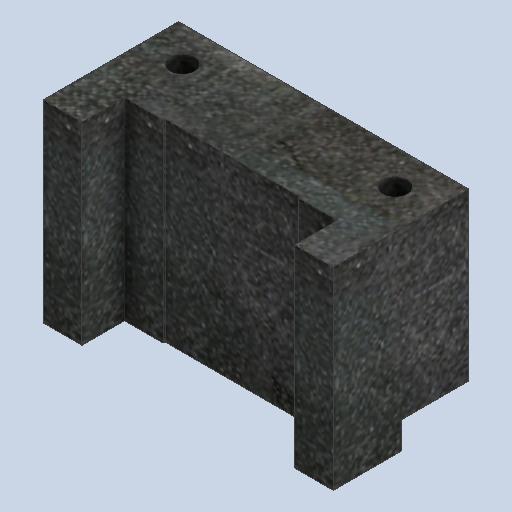
# Autodesk Inventor part: Lose backe
Saved by Autodesk Inventor 2023.2 (Build 272271000, 271)
## iProperties
Created: 2023-02-07
Part Number: Lose backe
Material: Steel
Document SubType Name: Modeling
Designer: Ayush
Density: 7.85 g/cm^3
Appearance: Plate
Author: Ayush
Autodesk Inventor part; units mm, degrees
ref_plane "YZ Plane" through (0, 0, 0) normal (1, 0, 0) x (0, 1, 0)
ref_plane "XZ Plane" through (0, 0, 0) normal (0, 1, 0) x (-1, 0, 0)
ref_plane "XY Plane" through (0, 0, 0) normal (0, 0, 1) x (1, 0, 0)
sketch "Sketch1" plane through (0, 0, 0) normal (0, 1, 0) x (-1, 0, 0)
  line L0 (-37.5, -17.5) -> (37.5, -17.5)
  line L1 (37.5, -17.5) -> (37.5, 17.5)
  line L2 (-37.5, 17.5) -> (-37.5, -17.5)
  line L3 (-37.5, -17.5) -> (37.5, 17.5) construction
  line L4 (37.5, -17.5) -> (-37.5, 17.5) construction
  line L5 (37.5, 17.5) -> (27.5, 17.5)
  line L6 (27.5, 17.5) -> (27.5, 6.5)
  line L7 (27.5, 6.5) -> (17.5, 6.5)
  line L8 (17.5, 6.5) -> (17.5, 6.0228)
  line L9 (17.5, 6.0228) -> (-17.5, 6.0228)
  line L10 (-17.5, 6.0228) -> (-17.5, 6.5)
  line L11 (-17.5, 6.5) -> (-27.5, 6.5)
  line L12 (-27.5, 6.5) -> (-27.5, 17.5)
  circle A0 centre (27.5, -8.5) radius 5.5
  circle A1 centre (-27.5, -8.5) radius 5.5
  circle A2 centre (0, -6.5) radius 5.5
  line L13 (37.5, 17.5) -> (27.5, 17.5)
  line L14 (-27.5, 17.5) -> (-37.5, 17.5)
  line L15 (-37.5, 1.5) -> (37.5, 1.5)
  line L16 (-37.5, 17.5) -> (-37.5, 1.5)
  line L17 (37.5, 1.5) -> (37.5, 17.5)
  line L18 (27.5, 17.5) -> (27.5, 6.5)
  line L19 (17.5, 6.5) -> (17.5, 6.0228)
  line L20 (-17.5, 6.0228) -> (-17.5, 6.5)
  line L21 (-27.5, 6.5) -> (-27.5, 17.5)
  line L22 (-37.5, 17.5) -> (-37.5, 1.5)
  point P0 (0, 0)
  point P1 (-32.5, 17.5)
  dimension "d0" = 75
  dimension "d1" = 35
  dimension "d2" = 10
  dimension "d3" = 11
  dimension "d4" = 10
  dimension "d5" = 35
  dimension "d6" = 10
  dimension "d7" = 11
  dimension "d8" = 11
  dimension "d10" = 11
  dimension "d12" = 27.5
  dimension "d13" = 27.5
  dimension "d41" = 16
  constraints: 46 end point, 7 perpendicular, 6 collinear, 4 parallel, 3 centre point, 3 horizontal, 3 midpoint, 2 point on line, 1 horizontal alignment, 1 vertical
  measures "d0" distance of L2.start L1.end
  measures "d1" distance of L1.end L0.end
  measures "d2" distance of L1.end L5.end
  measures "d3" distance of L5.end L6.end
  measures "d4" distance of L6.end L7.end
  measures "d5" distance of L8.end L9.end
  measures "d6" distance of L10.end L11.end
  measures "d7" diameter of A0
  measures "d8" diameter of A1
  measures "d10" diameter of A2
  measures "d12" horizontal distance of A1.centre A2.centre
  measures "d13" horizontal distance of A0.centre A2.centre
  measures "d41" distance from line of L15 point (-32.5, 17.5)
extrude "Extrusion1" add sketch "Sketch1" along normal blind 7
sketch "Sketch2" plane through (0, 7, 0) normal (0, 1, 0) x (1, 0, 0)
  line L0 (-37.5, 17.5) -> (-37.5, -17.5) projected
  line L1 (-37.5, -17.5) -> (-37.5, 17.5)
  line L2 (37.5, 17.5) -> (-37.5, 17.5) projected
  line L3 (-37.5, 17.5) -> (37.5, 17.5)
  line L4 (37.5, -17.5) -> (37.5, 17.5) projected
  line L5 (37.5, 17.5) -> (37.5, -17.5)
  line L6 (27.5, -17.5) -> (37.5, -17.5) projected
  line L7 (37.5, -17.5) -> (27.5, -17.5)
  line L8 (27.5, -6.5) -> (27.5, -17.5) projected
  line L9 (27.5, -17.5) -> (27.5, -6.5)
  line L10 (17.5, -6.5) -> (27.5, -6.5) projected
  line L11 (27.5, -6.5) -> (17.5, -6.5)
  line L12 (17.5, -6.0228) -> (17.5, -6.5) projected
  line L13 (17.5, -6.5) -> (17.5, -6.0228)
  line L14 (-17.5, -6.0228) -> (17.5, -6.0228) projected
  line L15 (17.5, -6.0228) -> (-17.5, -6.0228)
  line L16 (-17.5, -6.0228) -> (-17.5, -6.5)
  line L17 (-27.5, -6.5) -> (-17.5, -6.5) projected
  line L18 (-17.5, -6.5) -> (-27.5, -6.5)
  line L19 (-27.5, -17.5) -> (-27.5, -6.5) projected
  line L20 (-27.5, -6.5) -> (-27.5, -17.5)
  line L21 (-37.5, -17.5) -> (-27.5, -17.5) projected
  line L22 (-27.5, -17.5) -> (-37.5, -17.5)
  circle A0 centre (27.5, 8.5) radius 3.2
  circle A1 centre (-27.5, 8.5) radius 3.2
  circle A2 centre (0, 6.5) radius 5.5
  point P0 (0, 0)
  point P1 (-32.5, -17.5)
  dimension "d17" = 6.4
  dimension "d24" = 6.4
  dimension "d25" = 27.5
  dimension "d26" = 27.5
  dimension "d27" = 26
  dimension "d28" = 26
  dimension "d29" = 11
  dimension "d30" = 24
  constraints: 24 end point, 8 collinear, 3 centre point, 3 perpendicular, 1 midpoint, 1 point on line, 1 vertical
  measures "d17" diameter of A0
  measures "d24" diameter of A1
  measures "d25" horizontal distance of A1.centre point (0, 0)
  measures "d26" horizontal distance of A0.centre point (0, 0)
  measures "d27" distance from line of A1.centre L21
  measures "d28" distance from line of A0.centre L6
  measures "d29" diameter of A2
  measures "d30" vertical distance of A2.centre point (-32.5, -17.5)
extrude "Extrusion2" add sketch "Sketch2" along normal blind 13
sketch "Sketch3" plane through (0, 20, 0) normal (0, 1, 0) x (1, 0, 0)
  line L0 (-37.5, -17.5) -> (-27.5, -17.5) projected
  line L1 (-37.5, -17.5) -> (-27.5, -17.5)
  line L2 (-27.5, -17.5) -> (-27.5, -6.5) projected
  line L3 (-27.5, -17.5) -> (-27.5, -6.5)
  line L4 (-27.5, -6.5) -> (-17.5, -6.5) projected
  line L5 (-27.5, -6.5) -> (-17.5, -6.5)
  line L6 (-17.5, -6.5) -> (-17.5, -6.0228) projected
  line L7 (-17.5, -6.5) -> (-17.5, -6.0228)
  line L8 (-17.5, -6.0228) -> (17.5, -6.0228) projected
  line L9 (-17.5, -6.0228) -> (17.5, -6.0228)
  line L10 (17.5, -6.0228) -> (17.5, -6.5) projected
  line L11 (17.5, -6.0228) -> (17.5, -6.5)
  line L12 (17.5, -6.5) -> (27.5, -6.5) projected
  line L13 (17.5, -6.5) -> (27.5, -6.5)
  line L14 (27.5, -6.5) -> (27.5, -17.5) projected
  line L15 (27.5, -6.5) -> (27.5, -17.5)
  line L16 (27.5, -17.5) -> (37.5, -17.5) projected
  line L17 (27.5, -17.5) -> (37.5, -17.5)
  line L18 (37.5, 17.5) -> (-37.5, 17.5) projected
  line L19 (37.5, -17.5) -> (37.5, 17.5)
  line L20 (37.5, 17.5) -> (-37.5, 17.5)
  line L21 (-37.5, 17.5) -> (-37.5, -17.5) projected
  line L22 (-37.5, 17.5) -> (-37.5, -17.5)
  circle A0 centre (-27.5, 8.5) radius 3.2
  circle A1 centre (27.5, 8.5) radius 3.2
  point P0 (0, 0)
  point P1 (0, -6.0228)
  point P2 (0, -6.0228)
  dimension "d33" = 6.4
  dimension "d34" = 6.4
  dimension "d35" = 26
  dimension "d36" = 27.5
  dimension "d37" = 27.5
  constraints: 24 end point, 6 perpendicular, 5 collinear, 2 centre point, 2 midpoint, 1 horizontal, 1 horizontal alignment
  measures "d33" diameter of A0
  measures "d34" diameter of A1
  measures "d35" distance from line of A0.centre L0
  measures "d36" horizontal distance of point (0, -6.023) A0.centre
  measures "d37" horizontal distance of point (0, -6.023) A1.centre
extrude "Extrusion3" add sketch "Sketch3" along normal blind 23
sketch "Sketch5" plane through (0, 0, 0) normal (0, -1, 0) x (1, 0, 0)
  line L0 (37.5, 17.5) -> (37.5, -17.5) projected
  line L1 (37.5, 0) -> (-37.5, 0)
  line L2 (-37.5, -17.5) -> (-37.5, 17.5) projected
  line L3 (-37.5, 17.5) -> (-27.5, 17.5) projected
  line L4 (-37.5, 17.5) -> (-27.5, 17.5)
  line L5 (-27.5, 17.5) -> (-27.5, 6.5) projected
  line L6 (-27.5, 17.5) -> (-27.5, 6.5)
  line L7 (-27.5, 6.5) -> (-17.5, 6.5) projected
  line L8 (-27.5, 6.5) -> (-17.5, 6.5)
  line L9 (-17.5, 6.0228) -> (17.5, 6.0228) projected
  line L10 (-17.5, 6.5) -> (-17.5, 6.0228)
  line L11 (-17.5, 6.0228) -> (17.5, 6.0228)
  line L12 (17.5, 6.0228) -> (17.5, 6.5)
  line L13 (17.5, 6.5) -> (27.5, 6.5) projected
  line L14 (17.5, 6.5) -> (27.5, 6.5)
  line L15 (27.5, 6.5) -> (27.5, 17.5) projected
  line L16 (27.5, 6.5) -> (27.5, 17.5)
  line L17 (27.5, 17.5) -> (37.5, 17.5) projected
  line L18 (27.5, 17.5) -> (37.5, 17.5)
  line L19 (37.5, 17.5) -> (37.5, 0)
  point P0 (0, 0)
  constraints: 22 end point, 6 perpendicular, 4 collinear, 2 midpoint, 1 point on line
extrude "Extrusion4" add sketch "Sketch5" along normal blind 7
body "Solid1"
